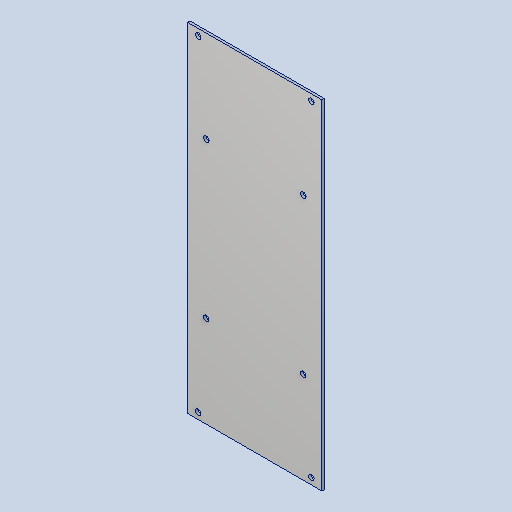
# Autodesk Inventor part: memesat shear panel type 2
Saved by Autodesk Inventor 2022 (Build 260153000, 153)
## iProperties
Created: 2020-02-20
Part Number: memesat shear panel type 2
Material: Aluminum 6061
Document SubType Name: Modeling
Designer: UGA SSRL
Density: 2.7 g/cm^3
Appearance: Aluminum - Flat
Mass: 25.6903 g
Surface Area: 110.966 cm^2
Volume: 9.51491 cm^3
Author: UGA SSRL
Autodesk Inventor part; units mm, degrees
ref_plane "YZ Plane" through (0, 0, 0) normal (1, 0, 0) x (0, 1, 0)
ref_plane "XZ Plane" through (0, 0, 0) normal (0, 1, 0) x (-1, 0, 0)
ref_plane "XY Plane" through (0, 0, 0) normal (0, 0, 1) x (1, 0, 0)
sketch "Sketch1" plane through (0, 0, 0) normal (0, 0, 1) x (1, 0, 0)
  line L0 (-41.5, 48) -> (41.5, 48)
  line L1 (41.5, 48) -> (41.5, -48)
  line L2 (41.5, -48) -> (-41.5, -48)
  line L3 (-41.5, -48) -> (-41.5, 48)
  point P0 (0, 0)
  dimension "d0" = 83
  dimension "d1" = 96
  dimension "d2" = 48
  dimension "d3" = 41.5
  constraints: 8 end point, 2 parallel, 1 horizontal, 1 perpendicular
  measures "d0" distance of L1.end L2.end
  measures "d1" distance of L0.end L1.end
  measures "d2" distance from line of L0 point (0, 0)
  measures "d3" distance from line of point (0, 0) L3
extrude "Extrusion1" add sketch "Sketch1" against normal blind 1.5
sketch "Sketch7" plane through (-41.5, 48, 0) normal (0, 1, 0) x (1, 0, 0)
  line L0 (0, 0) -> (83, 0) projected
  line L1 (83, 0) -> (83, 1.5) projected
  line L2 (0, 1.5) -> (83, 1.5) projected
  line L3 (0, 0) -> (0, 1.5) projected
  point P0 (41.5, 0)
extrude "Extrusion5" add sketch "Sketch7" along normal blind 56.75
sketch "Sketch8" plane through (-41.5, -48, 0) normal (0, -1, 0) x (1, 0, 0)
  line L0 (83, 0) -> (0, 0) projected
  line L1 (0, 0) -> (0, -1.5) projected
  line L2 (83, -1.5) -> (0, -1.5) projected
  line L3 (83, 0) -> (83, -1.5) projected
  point P0 (41.5, 0)
extrude "Extrusion6" add sketch "Sketch8" along normal blind 56.75
sketch "Sketch9" plane through (0, 0, 0) normal (0, 0, 1) x (1, 0, 0)
  circle A0 centre (35, -100.75) radius 3 projected
  circle A1 centre (-35, -100.75) radius 3 projected
  circle A2 centre (-30, -48) radius 3 projected
  circle A3 centre (30, -48) radius 3 projected
  circle A4 centre (30, 48) radius 3 projected
  circle A5 centre (-30, 48) radius 3 projected
  circle A6 centre (35, 100.75) radius 3 projected
  circle A7 centre (-35, 100.75) radius 3 projected
  point P0 (0, 0)
hole "Hole3" at (35, -100.75, 0) at (-35, -100.75, 0) at (30, -48, 0) at (-30, -48, 0) at (30, 48, 0) at (-30, 48, 0) at (35, 100.75, 0) at (-35, 100.75, 0) direction (0, 0, -1) diameter 3.454 end through all clearance for "Flat Head Machine Screw (82)" size "#4" standard "Ansi Unified Screw Threads"
equation "\"d2\" = 0.5 * d1"
equation "\"d3\" = 0.5 * d0"
body "Solid1"
